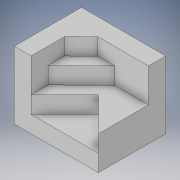
# Autodesk Inventor part: 零件19
Saved by Autodesk Inventor 2019 (Build 230136000, 136)
## iProperties
Created: 2020-09-18
Part Number: 零件19
Material: 一般
Document SubType Name: Modeling
Designer: jay
Density: 1 g/cm^3
Appearance: 預設
Author: jay
Autodesk Inventor part; units mm, degrees
ref_plane "YZ Plane" through (0, 0, 0) normal (1, 0, 0) x (0, 1, 0)
ref_plane "XZ Plane" through (0, 0, 0) normal (0, 1, 0) x (-1, 0, 0)
ref_plane "XY Plane" through (0, 0, 0) normal (0, 0, 1) x (1, 0, 0)
sketch "草圖1" plane through (0, 0, 0) normal (0, 0, 1) x (1, 0, 0)
  line L0 (0, 0) -> (50, 0)
  line L1 (50, 0) -> (50, 40)
  line L2 (50, 40) -> (0, 40)
  line L3 (0, 40) -> (0, 0)
  dimension "d0" = 50
  dimension "d1" = 40
  constraints: 8 end point, 2 parallel, 1 horizontal, 1 perpendicular
  measures "d0" distance of L1.end L2.end
  measures "d1" distance of L2.end L0.start
extrude "擠出1" add sketch "草圖1" along normal blind 40
sketch "草圖2" plane through (0, 40, 0) normal (0, 1, 0) x (1, 0, 0)
  line L0 (50, 0) -> (0, 0) projected
  line L1 (0, 0) -> (0, -40) projected
  line L2 (50, -40) -> (0, -40) projected
  line L3 (50, 0) -> (50, -40) projected
  line L4 (10, -40) -> (10, -20)
  line L5 (10, -20) -> (20, -10.2609)
  line L6 (20, -10.2609) -> (50, -10.2609)
  line L7 (50, 0) -> (50, -40) projected
  point P0 (0, 0)
  dimension "d4" = 10
  dimension "d5" = 10.2608
  dimension "d6" = 30
  dimension "d7" = 20
  constraints: 6 end point, 2 point on line, 1 perpendicular, 1 vertical
  measures "d4" distance between parallel lines of L1 L4
  measures "d5" distance between parallel lines of L0 L6
  measures "d6" distance from line of L3 L5.end
  measures "d7" distance from line of L2 L4.end
extrude "擠出2" cut sketch "草圖2" against normal blind 10 contours L3 L2 L4 L5 L6
sketch "草圖3" plane through (0, 30, 0) normal (0, 1, 0) x (1, 0, 0)
  line L0 (50, -10.2609) -> (50, -40) projected
  line L1 (20, -10.2609) -> (50, -10.2609) projected
  line L2 (10, -20) -> (20, -10.2609) projected
  line L3 (10, -40) -> (10, -20) projected
  line L4 (50, -40) -> (10, -40) projected
  line L5 (10, -29.7391) -> (30, -10.2609)
  point P0 (0, 0)
  dimension "d10" = 10
  constraints: 2 end point, 2 point on line, 1 parallel
  measures "d10" distance of L5.end L1.start
extrude "擠出3" cut sketch "草圖3" against normal blind 10 contours L0 L4 L3 L5 L1
sketch "草圖4" plane through (0, 20, 0) normal (0, 1, 0) x (1, 0, 0)
  line L0 (50, -10.2609) -> (50, -40) projected
  line L1 (30, -10.2609) -> (50, -10.2609) projected
  line L2 (10, -29.7391) -> (30, -10.2609) projected
  line L3 (10, -40) -> (10, -29.7391) projected
  line L4 (50, -40) -> (10, -40) projected
  line L5 (0, -40) -> (50, -40) projected
  line L6 (30, -20) -> (50, -40)
  line L7 (30, -20) -> (10, -40)
  point P0 (0, 0)
  dimension "d15" = 20
  constraints: 4 end point, 1 perpendicular
  measures "d15" distance from line of L0 L6.start
extrude "擠出4" cut sketch "草圖4" against normal blind 10 contours L4 L7 L6
